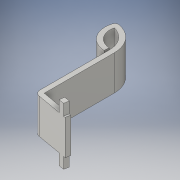
# Autodesk Inventor part: Lever
Saved by Autodesk Inventor 2016 (Build 200138000, 138)
## iProperties
Created: 2016-05-07
Part Number: Lever
Material: Stainless Steel
Document SubType Name: Modeling
Designer: agmle
Density: 8 g/cm^3
Appearance: Semi-Polished
Author: agmle
Autodesk Inventor part; units mm, degrees
ref_plane "YZ Plane" through (0, 0, 0) normal (1, 0, 0) x (0, 1, 0)
ref_plane "XZ Plane" through (0, 0, 0) normal (0, 1, 0) x (-1, 0, 0)
ref_plane "XY Plane" through (0, 0, 0) normal (0, 0, 1) x (1, 0, 0)
sketch "Sketch1" plane through (0, 0, 0) normal (0, 1, 0) x (-1, 0, 0)
  line L0 (0, 0) -> (4.2574, -0.7507)
  line L1 (4.8854, -1.4991) -> (4.8854, -10.87)
  line L2 (0, 0) -> (-0.1146, -0.65)
  line L3 (-0.1146, -0.65) -> (4.1428, -1.4007)
  line L4 (4.2254, -1.4991) -> (4.2254, -10.87)
  line L5 (4.8854, -7.3684) -> (4.2254, -7.3684) construction
  arc A0 (4.8854, -1.4991) -> (4.2574, -0.7507) centre (4.1254, -1.4991) ccw
  arc A1 (4.2254, -1.4991) -> (4.1428, -1.4007) centre (4.1254, -1.4991) ccw
  line L6 (0, 0) -> (9.7928, 0) construction
  arc A2 (4.2254, -10.87) -> (7.5579, -14.4878) centre (7.8554, -10.87) ccw
  arc A3 (4.8854, -10.87) -> (7.1313, -13.7504) centre (7.8554, -10.87) ccw
  arc A4 (7.1313, -13.7504) -> (5.1401, -11.0799) centre (5.0441, -13.2291) ccw
  line L7 (7.1313, -13.7504) -> (6.9714, -14.3907) construction
  line L8 (7.1313, -13.7504) -> (7.7714, -13.9113) construction
  line L9 (5.1401, -11.0799) -> (5.1689, -10.4206)
  arc A5 (7.5579, -14.4878) -> (5.1689, -10.4206) centre (5.0441, -13.2291) ccw
  line L10 (7.8554, -14.5) -> (1.0376, -14.5) construction
  line L11 (7.8554, -14.5) -> (7.8554, -9.8671) construction
  dimension "d0" = 0.66
  dimension "d2" = 10
  dimension "d3" = 0.1
  dimension "d4" = 14.5
  dimension "d5" = 5
  dimension "d6" = 3.63
  dimension "d8" = 2.5
  dimension "d9" = 4.0794
  constraints: 24 end point, 14 point on circle, 10 tangent, 6 centre point, 4 equal length, 3 coincident, 3 perpendicular, 3 point on line, 3 vertical, 1 horizontal, 1 parallel
  measures "d0" distance of L5.start L5.end
  measures "d2" angle of L6 L0
  measures "d3" radius of A1
  measures "d4" distance between parallel lines of L6 L10
  measures "d5" distance from line of L2.end L1
  measures "d6" distance between parallel lines of L4 L11
  measures "d8" angle of L1 L9
  measures "d9" distance from line of L10 L9.end
extrude "Extrusion1" add sketch "Sketch1" along normal blind 4.7
fillet "Fillet1" radius 0.5 1 edges at (-7.5579, 2.35, -14.4878)
sketch "Sketch2" plane through (0, 0, 0) normal (-0.1736482, 0, 0.9848078) x (0.9848078, 0, 0.1736482)
  line L0 (-4.323, 4.7) -> (0, 4.7) projected
  line L1 (0, 0) -> (-4.323, 0) projected
  line L2 (-1, 4.7) -> (-0.25, 4.7)
  line L3 (-0.25, 4.7) -> (-0.25, 6.2)
  line L4 (-0.25, 6.2) -> (-1, 6.2)
  line L5 (-1, 6.2) -> (-1, 4.7)
  line L6 (-1, 0) -> (-0.25, 0)
  line L7 (-0.25, 0) -> (-0.25, -1.5)
  line L8 (-0.25, -1.5) -> (-1, -1.5)
  line L9 (-1, -1.5) -> (-1, 0)
  line L10 (0, 0) -> (0, 4.7) projected
  dimension "d13" = 1.5
  dimension "d14" = 0.75
  dimension "d15" = 0.25
  constraints: 16 end point, 4 parallel, 4 point on line, 2 horizontal, 2 perpendicular, 1 collinear
  measures "d13" distance of L6.end L7.end
  measures "d14" distance of L7.end L8.end
  measures "d15" distance between parallel lines of L10 L3
extrude "Extrusion2" add sketch "Sketch2" against normal up to surface (0.66 mm away)
body "Solid1"
